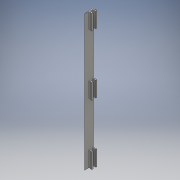
# Autodesk Inventor part: LedStripHolder
Saved by Autodesk Inventor 2016 (Build 200138000, 138)
## iProperties
Created: 2015-05-25
Part Number: LedStripHolder
Material: Generic
Document SubType Name: Modeling
Designer: Jack
Density: 1 g/cm^3
Appearance: Default
Author: Jack
Autodesk Inventor part; units mm, degrees
ref_plane "YZ Plane" through (0, 0, 0) normal (1, 0, 0) x (0, 1, 0)
ref_plane "XZ Plane" through (0, 0, 0) normal (0, 1, 0) x (-1, 0, 0)
ref_plane "XY Plane" through (0, 0, 0) normal (0, 0, 1) x (1, 0, 0)
sketch "Sketch1" plane through (0, 0, 0) normal (0, 0, 1) x (1, 0, 0)
  line L0 (0, 0) -> (-1.6865, 12)
  line L1 (-1.6865, 12) -> (0, 12)
  line L2 (0, 12) -> (0, 0)
  dimension "d0" = 8
  dimension "d1" = 12
  constraints: 6 end point, 1 horizontal, 1 perpendicular
  measures "d0" angle of L2 L0
  measures "d1" distance of L1.end L0.start
extrude "Extrusion1" add sketch "Sketch1" along normal blind 175
sketch "Sketch2" plane through (0, 0, 175) normal (0, 0, 1) x (1, 0, 0)
  line L0 (0, 0) -> (0, 12) projected
  line L1 (0, 12) -> (-1.6865, 12) projected
  line L2 (0, 12) -> (2, 12)
  line L3 (2, 12) -> (2.3, 12.3)
  line L4 (2.3, 12.3) -> (4, 12.3)
  line L5 (4, 12.3) -> (4, 10.8)
  line L6 (4, 10.8) -> (0, 10.8)
  line L7 (0, 7.2) -> (4, 7.2)
  line L8 (4, 7.2) -> (4, 5.7)
  line L9 (4, 5.7) -> (2.3, 5.7)
  line L10 (2.3, 5.7) -> (2, 6)
  line L11 (2, 6) -> (0, 6)
  dimension "d4" = 2
  dimension "d5" = 4
  dimension "d6" = 135
  dimension "d9" = 135
  dimension "d17" = 6
  dimension "d18" = 6.6
  dimension "d19" = 1.2
  constraints: 20 end point, 5 perpendicular, 4 equal length, 3 horizontal, 3 point on line, 1 collinear, 1 midpoint
  measures "d4" distance of L2.start L2.end
  measures "d5" distance of L5.end L6.end
  measures "d6" angle of L3 L2
  measures "d9" angle of L11 L10
  measures "d17" distance between parallel lines of L2 L11
  measures "d18" distance between parallel lines of L9 L4
  measures "d19" distance between parallel lines of L2 L6
extrude "Extrusion2" add sketch "Sketch2" against normal blind 20
pattern_linear "Rectangular Pattern1" count 3 spacing 77.5 along (0, 0, -1) of "Extrusion2"
body "Solid1"
